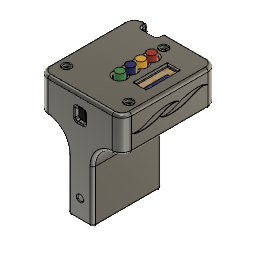
RangeFinderCase (Autodesk Fusion 360 design; units mm, degrees)
Autodesk Fusion 360 part; units mm, degrees
(part 1 of 2)
sketch "Sketch1" plane through (0, 0, 0) normal (0, 0, 1) x (1, 0, 0)
  line L0 (-22.5, 32.5) -> (22.5, 32.5) construction
  line L1 (22.5, 32.5) -> (22.5, -32.5) construction
  line L2 (22.5, -32.5) -> (-22.5, -32.5) construction
  line L3 (-22.5, -32.5) -> (-22.5, 32.5) construction
  circle A0 centre (-22.5, -32.5) radius 1.6
  circle A1 centre (-22.5, 32.5) radius 1.6 construction
  circle A2 centre (22.5, 32.5) radius 1.6 construction
  circle A3 centre (22.5, -32.5) radius 1.6
  line L4 (0, 32.5) -> (0, -32.5) construction
  circle A4 centre (-21.59, -29.21) radius 0.5 construction
  circle A5 centre (21.59, -29.21) radius 0.5 construction
  circle A6 centre (-21.59, 29.21) radius 0.5 construction
  circle A7 centre (21.59, 29.21) radius 0.5 construction
  line L5 (-21.59, 29.21) -> (-21.59, -29.21) construction
  line L6 (-21.59, -29.21) -> (21.59, -29.21) construction
  line L7 (21.59, -29.21) -> (21.59, 29.21) construction
  line L8 (21.59, 29.21) -> (-21.59, 29.21) construction
  line L9 (-21.59, 29.21) -> (21.59, -29.21) construction
  line L10 (21.59, 29.21) -> (-21.59, -29.21) construction
  circle A8 centre (1.27, 13.97) radius 1.6
  line L11 (25.25, 19.05) -> (-25.25, 19.05)
  line L12 (-25.25, 19.05) -> (-25.25, -35.25)
  line L13 (-25.25, -35.25) -> (25.25, -35.25)
  line L14 (25.25, -35.25) -> (25.25, 19.05)
  line L15 (25.25, 19.05) -> (-25.25, -35.25) construction
  line L16 (-25.25, 19.05) -> (25.25, -35.25) construction
  line L17 (-22.5, -32.5) -> (-25.25, -32.5) construction
  line L18 (-22.5, -32.5) -> (-22.5, -35.25) construction
  line L19 (20.32, 5.08) -> (12.7, 5.08)
  line L20 (12.7, 5.08) -> (12.7, -17.78)
  line L21 (12.7, -17.78) -> (20.32, -17.78)
  line L22 (20.32, -17.78) -> (20.32, 5.08)
  line L23 (16.51, 5.08) -> (16.51, -17.78) construction
  circle A9 centre (2.54, -19.05) radius 3.05
  circle A10 centre (2.54, -11.43) radius 3.05
  circle A11 centre (2.54, -3.81) radius 3.05
  circle A12 centre (2.54, 3.81) radius 3.05
  line L24 (2.54, -19.05) -> (2.54, -11.43) construction
  line L25 (2.54, -11.43) -> (2.54, -3.81) construction
  line L26 (2.54, -3.81) -> (2.54, 3.81) construction
  line L27 (-5.08, 17.78) -> (-22.86, 17.78)
  line L28 (-22.86, 17.78) -> (-22.86, -17.78)
  line L29 (-22.86, -17.78) -> (-5.08, -17.78)
  line L30 (-5.08, -17.78) -> (-5.08, 17.78)
  point P0 (0, -8.1)
  dimension "d15" = 45
  dimension "d16" = 65
  dimension "d18" = 3.2
  dimension "d47" = 58.42
  dimension "d48" = 43.18
  dimension "d49" = 1
  dimension "d50" = 43.18
  dimension "d51" = 22.86
  dimension "d52" = 50.5
  dimension "d53" = 5.08
  dimension "d68" = 7.62
  dimension "d69" = 22.86
  dimension "d71" = 11.43
  dimension "d74" = 6.1
  dimension "d75" = 7.62
  dimension "d76" = 10.16
  dimension "d80" = 17.78
  dimension "d81" = 35.56
  dimension "d83" = 11.43
  dimension "d182" = 1.27
  dimension "d188" = 1.27
  dimension "d189" = 19.05
  constraint horizontal L0
  constraint vertical L1
  constraint horizontal L2
  constraint vertical L3
  constraint coincident L2.end L3.start
  constraint coincident L0.start L3.end
  constraint coincident L0.end L1.start
  constraint coincident L1.end L2.start
  constraint equal A1 A2
  constraint equal A0 A1
  constraint equal A1 A3
  constraint midpoint L0 L4.start
  constraint midpoint L2 L4.end
  constraint midpoint origin L4
  constraint coincident A6.centre L5.start
  constraint coincident A4.centre L5.end
  constraint coincident A5.centre L6.end
  constraint coincident A7.centre L7.end
  constraint horizontal L8
  constraint vertical L5
  constraint equal L6 L8
  constraint equal L5 L7
  constraint midpoint origin L9
  constraint equal A6 A7
  constraint equal A4 A6
  constraint equal A5 A6
  constraint equal A1 A8
  constraint horizontal L11
  constraint perpendicular L11 L12
  constraint parallel L11 L13
  constraint parallel L12 L14
  constraint coincident L15 P0
  constraint coincident L16 P0
  constraint coincident L4 P0
  constraint coincident L12 L17.end
  constraint perpendicular L12 L17
  constraint coincident L13 L18.end
  constraint perpendicular L13 L18
  constraint equal L17 L18
  constraint horizontal L19
  constraint vertical L20
  constraint horizontal L21
  constraint vertical L22
  constraint midpoint L19 L23.start
  constraint midpoint L21 L23.end
  constraint coincident A9.centre L24.start
  constraint coincident A10.centre L24.end
  constraint vertical L24
  constraint coincident A11.centre L25.end
  constraint parallel L24 L25
  constraint coincident A12.centre L26.end
  constraint parallel L25 L26
  constraint equal L24 L25
  constraint equal L24 L26
  constraint equal A9 A10
  constraint equal A10 A11
  constraint equal A11 A12
  constraint horizontal L27
  constraint vertical L28
  constraint horizontal L29
  constraint vertical L30
  measures "d15" distance of L1.end L2.end
  measures "d16" distance of L0.start L2.end
  measures "d18" diameter of A1
  measures "d47" distance of A5.centre A7.centre
  measures "d48" distance of A4.centre A5.centre
  measures "d49" diameter of A6
  measures "d50" distance of L6 A8.centre
  measures "d51" distance of L5 A8.centre
  measures "d52" distance of L12.end L13.end
  measures "d53" distance of A8.centre L11
  measures "d68" distance of L19.start L19.end
  measures "d69" distance of L19.start L21.end
  measures "d71" distance of L6 L21
  measures "d74" diameter of A9
  measures "d75" distance of A9.centre A10.centre
  measures "d76" distance of L6 A9.centre
  measures "d80" distance of L28.end L29.end
  measures "d81" distance of L27.end L28.end
  measures "d83" distance of L6 L29
  measures "d182" distance of L7 L22
  measures "d188" distance of L5 L28
  measures "d189" distance of L7 L24
extrude "Extrude5" add sketch "Sketch1" along normal blind 1.2 contours L11 L12 L13 L14 | L19 L20 L21 L22 | A9 | A10 | A11 | A12 | L27 L28 L29 L30 makes body 1
sketch "Sketch5" plane through (0, -35.25, 0) normal (0, -1, 0) x (1, 0, 0)
  line L0 (-25.25, 0) -> (25.25, 0)
  line L1 (25.25, 0) -> (25.25, 1.2)
  line L2 (25.25, 1.2) -> (-25.25, 1.2)
  line L3 (-25.25, 1.2) -> (-25.25, 0)
  line L4 (13, 5.7) -> (-13, 5.7)
  line L5 (-13, 5.7) -> (-13, -12.3)
  line L6 (-13, -12.3) -> (13, -12.3)
  line L7 (13, -12.3) -> (13, 5.7)
  line L8 (13, 5.7) -> (-13, -12.3) construction
  line L9 (-13, 5.7) -> (13, -12.3) construction
  line L10 (0, -3.3) -> (0, 0) construction
  point P0 (0, -3.3)
  dimension "d56" = 26
  dimension "d57" = 18
  dimension "d58" = 4.5
  constraint horizontal L4
  constraint perpendicular L4 L5
  constraint parallel L4 L6
  constraint parallel L5 L7
  constraint coincident L8 P0
  constraint coincident L9 P0
  constraint coincident P0 L10.start
  constraint coincident L10.end origin
  constraint vertical L10
  measures "d56" distance of L4.start L4.end
  measures "d57" distance of L4.end L5.end
  measures "d58" distance of L2 L4
extrude "Extrude6" add sketch "Sketch5" along normal blind 5 contours L0 L2 L5 L7 | L0 L5 L6 L7 | L2 L4 L5 L7 bodies 1
sketch "Sketch6" plane through (0, -40.25, 0) normal (0, -1, 0) x (1, 0, 0)
  line L0 (13, -12.3) -> (13, 5.7)
  line L1 (13, 5.7) -> (-13, 5.7)
  line L2 (-13, 5.7) -> (-13, -12.3)
  line L3 (-13, -12.3) -> (13, -12.3)
  line L4 (0, 5.7) -> (0, -12.3) construction
  line L5 (-13, -3.3) -> (13, -3.3) construction
  line L6 (1.5, -0.8) -> (-1.5, -0.8)
  line L7 (-1.5, -0.8) -> (-1.5, -5.8)
  line L8 (-1.5, -5.8) -> (1.5, -5.8)
  line L9 (1.5, -5.8) -> (1.5, -0.8)
  line L10 (1.5, -0.8) -> (-1.5, -5.8) construction
  line L11 (-1.5, -0.8) -> (1.5, -5.8) construction
  point P0 (0, -3.3)
  dimension "d61" = 5
  dimension "d62" = 3
  constraint midpoint L1 L4.start
  constraint midpoint L3 L4.end
  constraint midpoint L2 L5.start
  constraint midpoint L0 L5.end
  constraint horizontal L6
  constraint perpendicular L6 L7
  constraint parallel L6 L8
  constraint parallel L7 L9
  constraint coincident L10 P0
  constraint coincident L11 P0
  constraint midpoint L4 P0
  measures "d61" distance of L6.start L8.end
  measures "d62" distance of L6.start L6.end
extrude "Extrude7" cut sketch "Sketch6" against normal blind 0.1 contours L6 L7 L8 L9 bodies 1
sketch "Sketch7" plane through (0, 0, 1.2) normal (0, 0, 1) x (-1, 0, 0)
  circle A0 centre (-1.27, -13.97) radius 1.6
  circle A1 centre (-22.5, 32.5) radius 1.6
  circle A2 centre (22.5, 32.5) radius 1.6
  line L0 (-25.25, 35.25) -> (-25.25, -19.05)
  line L1 (-25.25, -19.05) -> (25.25, -19.05)
  line L2 (25.25, -19.05) -> (25.25, 35.25)
  line L3 (25.25, 35.25) -> (13, 35.25)
  line L4 (13, 35.25) -> (-13, 35.25)
  line L5 (-13, 35.25) -> (-25.25, 35.25)
  circle A3 centre (-1.27, -13.97) radius 2.7
  circle A4 centre (22.5, 32.5) radius 2.7
  circle A5 centre (-22.5, 32.5) radius 2.7
  dimension "d65" = 5.4
  constraint concentric A0 A3
  constraint concentric A2 A4
  constraint concentric A1 A5
  constraint equal A4 A5
  constraint equal A3 A4
  measures "d65" diameter of A4
extrude "Extrude8" add sketch "Sketch7" along normal blind 6 contours A3 | A4 | A5 bodies 1
extrude "Extrude9" add sketch "Sketch1" along normal up to surface (3.7 mm away) contours L19 L20 L21 L22 bodies 1
extrude "Extrude10" add sketch "Sketch1" along normal up to surface (13.2 mm away) contours A9 | A10 | A11 | A12 bodies 1
extrude "Extrude11" add sketch "Sketch1" along normal up to surface (5.7 mm away) contours L27 L28 L29 L30 bodies 1
sketch "Sketch8" plane through (0, 17.78, 0) normal (0, 1, 0) x (-1, 0, 0)
  line L0 (5.08, 1.2) -> (22.86, 1.2)
  line L1 (22.86, 1.2) -> (22.86, 5.7)
  line L2 (22.86, 5.7) -> (5.08, 5.7)
  line L3 (5.08, 5.7) -> (5.08, 1.2)
  line L4 (18.47, 7.7) -> (9.47, 7.7)
  line L5 (9.47, 7.7) -> (9.47, 4.7)
  line L6 (9.47, 4.7) -> (18.47, 4.7)
  line L7 (18.47, 4.7) -> (18.47, 7.7)
  line L8 (18.47, 7.7) -> (9.47, 4.7) construction
  line L9 (9.47, 7.7) -> (18.47, 4.7) construction
  line L10 (13.97, 5.7) -> (13.97, 1.2) construction
  point P0 (13.97, 6.2)
  dimension "d86" = 3.5
  dimension "d87" = 9
  dimension "d88" = 3
  constraint horizontal L4
  constraint perpendicular L4 L5
  constraint parallel L4 L6
  constraint parallel L5 L7
  constraint coincident L8 P0
  constraint coincident L9 P0
  constraint midpoint L2 L10.start
  constraint midpoint L0 L10.end
  constraint coincident P0 L10
  measures "d86" distance of L0 L6
  measures "d87" distance of L4.start L4.end
  measures "d88" distance of L4.start L6.end
extrude "Extrude12" add sketch "Sketch8" along normal blind 0.5 and the other way blind 6 contours L2 L4 L5 L7 | L2 L5 L6 L7 bodies 1
sketch "Sketch9" plane through (0, 0, 0) normal (0, 0, -1) x (1, 0, 0)
  circle A0 centre (22.5, 32.5) radius 1.6
  circle A1 centre (1.27, -13.97) radius 1.6
  circle A2 centre (-22.5, 32.5) radius 1.6
  line L0 (25.25, -19.05) -> (25.25, 35.25)
  line L1 (25.25, 35.25) -> (13, 35.25)
  line L2 (13, 35.25) -> (-13, 35.25)
  line L3 (-13, 35.25) -> (-25.25, 35.25)
  line L4 (-25.25, 35.25) -> (-25.25, -19.05)
  line L5 (-25.25, -19.05) -> (25.25, -19.05)
  circle A3 centre (-22.5, 32.5) radius 2
  circle A4 centre (-22.5, 32.5) radius 4
  circle A5 centre (22.5, 32.5) radius 2
  circle A6 centre (22.5, 32.5) radius 4
  circle A7 centre (1.27, -13.97) radius 2
  circle A8 centre (1.27, -13.97) radius 4
  line L6 (27.25, -21.05) -> (-27.25, -21.05)
  line L7 (-27.25, -21.05) -> (-27.25, 42.25)
  line L8 (-27.25, 42.25) -> (27.25, 42.25)
  line L9 (27.25, 42.25) -> (27.25, -21.05)
  line L10 (0, -21.05) -> (0, -19.05) construction
  line L11 (27.25, 10.6) -> (25.25, 10.6) construction
  line L12 (-27.25, 10.6) -> (-25.25, 10.6) construction
  line L13 (0, 42.25) -> (0, 40.25) construction
  line L14 (-13, 40.25) -> (13, 40.25) construction
  dimension "d93" = 4
  dimension "d94" = 2
  dimension "d95" = 2
  constraint concentric A2 A3
  constraint concentric A3 A4
  constraint concentric A0 A5
  constraint concentric A0 A6
  constraint concentric A1 A7
  constraint concentric A7 A8
  constraint equal A3 A5
  constraint equal A3 A7
  constraint equal A4 A8
  constraint equal A4 A6
  constraint horizontal L6
  constraint vertical L7
  constraint horizontal L8
  constraint vertical L9
  constraint midpoint L6 L10.start
  constraint coincident L5 L10.end
  constraint perpendicular L5 L10
  constraint midpoint L9 L11.start
  constraint coincident L0 L11.end
  constraint perpendicular L0 L11
  constraint midpoint L7 L12.start
  constraint coincident L4 L12.end
  constraint perpendicular L4 L12
  constraint midpoint L8 L13.start
  constraint perpendicular L8 L13
  constraint coincident L13.end L14
  constraint equal L11 L13
  constraint equal L11 L12
  constraint equal L10 L11
  measures "d93" diameter of A3
  measures "d94" distance of A3 A4
  measures "d95" distance of L11.start L11.end
extrude "Extrude13" add sketch "Sketch9" along normal up to surface (13.3 mm away) separate body contours L0 L1 A6 | L0 L1 A6 | L3 L4 A4 | L3 L4 A4 | A8 makes body 2 at (26.4801, -32.8983, -8.8667) makes body 3 at (-18.5199, -32.8983, -8.8667) makes body 4 at (5.265, 14.1694, -8.8667)
sketch "Sketch10" plane through (0, 0, -13.3) normal (0, 0, -1) x (1, 0, 0)
  circle A0 centre (1.27, -13.97) radius 2
  circle A1 centre (1.27, -13.97) radius 4
  line L0 (28.25, -22.05) -> (-28.25, -22.05)
  line L1 (-28.25, -22.05) -> (-28.25, 43.25)
  line L2 (-28.25, 43.25) -> (28.25, 43.25)
  line L3 (28.25, 43.25) -> (28.25, -22.05)
  circle A2 centre (22.5, 32.5) radius 1.6
  circle A3 centre (1.27, -13.97) radius 1.6
  circle A4 centre (-22.5, 32.5) radius 1.6
  line L4 (25.25, -19.05) -> (25.25, 35.25)
  line L5 (25.25, 35.25) -> (13, 35.25)
  line L6 (13, 35.25) -> (-13, 35.25)
  line L7 (-13, 35.25) -> (-25.25, 35.25)
  line L8 (-25.25, 35.25) -> (-25.25, -19.05)
  line L9 (-25.25, -19.05) -> (25.25, -19.05)
  line L10 (-13, 35.25) -> (13, 35.25)
  line L11 (13, 35.25) -> (13, 40.25)
  line L12 (13, 40.25) -> (-13, 40.25)
  line L13 (-13, 40.25) -> (-13, 35.25)
  line L14 (28.25, 10.6) -> (25.25, 10.6) construction
  line L15 (-28.25, 10.6) -> (-25.25, 10.6) construction
  line L16 (0, -22.05) -> (0, -19.05) construction
  line L17 (0, 43.25) -> (0, 40.25) construction
  dimension "d98" = 3
  constraint horizontal L0
  constraint vertical L1
  constraint horizontal L2
  constraint vertical L3
  constraint midpoint L3 L14.start
  constraint coincident L4 L14.end
  constraint perpendicular L4 L14
  constraint midpoint L1 L15.start
  constraint coincident L8 L15.end
  constraint perpendicular L8 L15
  constraint midpoint L0 L16.start
  constraint coincident L9 L16.end
  constraint perpendicular L9 L16
  constraint midpoint L2 L17.start
  constraint coincident L12 L17.end
  constraint perpendicular L12 L17
  constraint equal L14 L16
  constraint equal L14 L17
  constraint equal L14 L15
  measures "d98" distance of L14.start L14.end
extrude "Extrude14" add sketch "Sketch10" along normal blind 2 contours A0 | A1 | L0 L1 L2 L3 | A2 | A3 | A4 | L4 L5 L6 L7 L8 L9 L10 | L6 L10 L11 L12 L13 bodies 2 3 4
fillet "Fillet4" radius 5 4 edges at (-28.25, -43.25, -14.3) (28.25, -43.25, -14.3) (28.25, 22.05, -14.3) (-28.25, 22.05, -14.3) on bodies 2
sketch "Sketch11" plane through (0, 0, -15.3) normal (0, 0, -1) x (1, 0, 0)
  line L0 (23.25, 43.25) -> (-23.25, 43.25)
  line L1 (-28.25, 38.25) -> (-28.25, -17.05)
  line L2 (-23.25, -22.05) -> (23.25, -22.05)
  line L3 (28.25, -17.05) -> (28.25, 38.25)
  arc A0 (-28.25, -17.05) -> (-23.25, -22.05) centre (-23.25, -17.05) ccw
  arc A1 (23.25, -22.05) -> (28.25, -17.05) centre (23.25, -17.05) ccw
  arc A2 (28.25, 38.25) -> (23.25, 43.25) centre (23.25, 38.25) ccw
  arc A3 (-23.25, 43.25) -> (-28.25, 38.25) centre (-23.25, 38.25) ccw
  line L4 (30.25, -17.05) -> (30.25, 38.25)
  arc A4 (30.25, 38.25) -> (23.25, 45.25) centre (23.25, 38.25) ccw
  line L5 (23.25, 45.25) -> (-23.25, 45.25)
  arc A5 (-23.25, 45.25) -> (-30.25, 38.25) centre (-23.25, 38.25) ccw
  line L6 (-30.25, 38.25) -> (-30.25, -17.05)
  arc A6 (-30.25, -17.05) -> (-23.25, -24.05) centre (-23.25, -17.05) ccw
  line L7 (-23.25, -24.05) -> (23.25, -24.05)
  arc A7 (23.25, -24.05) -> (30.25, -17.05) centre (23.25, -17.05) ccw
  dimension "d101" = 2
extrude "Extrude15" add sketch "Sketch11" against normal up to surface (23.5 mm away) bodies 2
sketch "Sketch12" plane through (0, 24.05, 0) normal (0, 1, 0) x (-1, 0, 0)
  line L0 (23.25, 8.2) -> (-23.25, 8.2)
  line L1 (-23.25, 8.2) -> (-23.25, -15.3)
  line L2 (-23.25, -15.3) -> (23.25, -15.3)
  line L3 (23.25, -15.3) -> (23.25, 8.2)
  line L4 (9.47, 4.7) -> (18.47, 4.7)
  line L5 (18.47, 4.7) -> (18.47, 7.7)
  line L6 (18.47, 7.7) -> (9.47, 7.7)
  line L7 (9.47, 7.7) -> (9.47, 4.7)
  line L8 (9.47, 7.7) -> (18.47, 4.7) construction
  line L9 (18.47, 7.7) -> (9.47, 4.7) construction
  line L10 (19.97, 9.45) -> (7.97, 9.45)
  line L11 (7.97, 9.45) -> (7.97, 2.95)
  line L12 (7.97, 2.95) -> (19.97, 2.95)
  line L13 (19.97, 2.95) -> (19.97, 9.45)
  line L14 (19.97, 9.45) -> (7.97, 2.95) construction
  line L15 (7.97, 9.45) -> (19.97, 2.95) construction
  point P0 (13.97, 6.2)
  point P1 (13.97, 6.2)
  dimension "d106" = 6.5
  dimension "d107" = 12
  constraint coincident L6.end L7.start
  constraint coincident L4.end L5.start
  constraint coincident L5.end L6.start
  constraint coincident L4.start L7.end
  constraint coincident L8 P1
  constraint coincident L9 P1
  constraint horizontal L10
  constraint perpendicular L10 L11
  constraint parallel L10 L12
  constraint parallel L11 L13
  constraint coincident L14 P1
  constraint coincident L15 P1
  constraint coincident P1 P0
  measures "d106" distance of L10.start L12.end
  measures "d107" distance of L11.end L12.end
extrude "Extrude16" cut sketch "Sketch12" against normal blind 2 contours L0 L11 L12 L13 | L0 L10 L11 L13 | L4 L5 L6 L7 bodies 2
fillet "Fillet5" radius 2 2 edges at (-19.97, 23.05, 2.95) (-7.97, 23.05, 2.95) on bodies 2
sketch "Sketch13" plane through (0, 0, 8.2) normal (0, 0, 1) x (-1, 0, 0)
  line L0 (-23.25, 43.25) -> (23.25, 43.25)
  arc A0 (28.25, 38.25) -> (23.25, 43.25) centre (23.25, 38.25) ccw
  line L1 (28.25, 38.25) -> (28.25, -17.05)
  arc A1 (23.25, -22.05) -> (28.25, -17.05) centre (23.25, -17.05) ccw
  line L2 (7.97, -22.05) -> (-23.25, -22.05)
  arc A2 (-28.25, -17.05) -> (-23.25, -22.05) centre (-23.25, -17.05) ccw
  line L3 (-28.25, -17.05) -> (-28.25, 38.25)
  arc A3 (-23.25, 43.25) -> (-28.25, 38.25) centre (-23.25, 38.25) ccw
  line L4 (-30.25, 38.25) -> (-30.25, -17.05)
  arc A4 (-30.25, -17.05) -> (-23.25, -24.05) centre (-23.25, -17.05) ccw
  line L5 (19.97, -24.05) -> (23.25, -24.05)
  arc A5 (23.25, -24.05) -> (30.25, -17.05) centre (23.25, -17.05) ccw
  line L6 (30.25, -17.05) -> (30.25, 38.25)
  arc A6 (30.25, 38.25) -> (23.25, 45.25) centre (23.25, 38.25) ccw
  line L7 (23.25, 45.25) -> (-23.25, 45.25)
  arc A7 (-23.25, 45.25) -> (-30.25, 38.25) centre (-23.25, 38.25) ccw
  line L8 (-12.7, 17.78) -> (-20.32, 17.78)
  line L9 (-20.32, 17.78) -> (-20.32, -5.08)
  line L10 (-20.32, -5.08) -> (-12.7, -5.08)
  line L11 (-12.7, -5.08) -> (-12.7, 17.78)
  circle A8 centre (-2.54, 19.05) radius 3.05 construction
  circle A9 centre (-2.54, 11.43) radius 3.05 construction
  circle A10 centre (-2.54, 3.81) radius 3.05 construction
  circle A11 centre (-2.54, -3.81) radius 3.05 construction
  circle A12 centre (-2.54, 19.05) radius 4.06
  circle A13 centre (-2.54, 11.43) radius 4.06
  circle A14 centre (-2.54, 3.81) radius 4.06
  circle A15 centre (-2.54, -3.81) radius 4.06
  line L12 (-2.54, 15.49) -> (-2.54, 14.99) construction
  line L13 (19.97, -22.05) -> (19.97, -24.05)
  line L14 (-23.25, -24.05) -> (7.97, -24.05)
  line L15 (7.97, -24.05) -> (7.97, -22.05)
  line L16 (23.25, -22.05) -> (19.97, -22.05)
  line L17 (11.2, -21.95) -> (-23.25, -21.95)
  arc A16 (-28.15, -17.05) -> (-23.25, -21.95) centre (-23.25, -17.05) ccw
  line L18 (-28.15, -17.05) -> (-28.15, 38.25)
  arc A17 (-23.25, 43.15) -> (-28.15, 38.25) centre (-23.25, 38.25) ccw
  line L19 (-23.25, 43.15) -> (23.25, 43.15)
  arc A18 (28.15, 38.25) -> (23.25, 43.15) centre (23.25, 38.25) ccw
  line L20 (28.15, 38.25) -> (28.15, -17.05)
  arc A19 (23.25, -21.95) -> (28.15, -17.05) centre (23.25, -17.05) ccw
  line L21 (8.38, -20.05) -> (-23.25, -20.05)
  arc A20 (-26.25, -17.05) -> (-23.25, -20.05) centre (-23.25, -17.05) ccw
  line L22 (-26.25, -17.05) -> (-26.25, 38.25)
  arc A21 (-23.25, 41.25) -> (-26.25, 38.25) centre (-23.25, 38.25) ccw
  line L23 (-23.25, 41.25) -> (23.25, 41.25)
  arc A22 (26.25, 38.25) -> (23.25, 41.25) centre (23.25, 38.25) ccw
  line L24 (26.25, 38.25) -> (26.25, -17.05)
  arc A23 (23.25, -20.05) -> (26.25, -17.05) centre (23.25, -17.05) ccw
  line L25 (8.38, -20.05) -> (23.25, -20.05)
  line L26 (11.2, -21.95) -> (23.25, -21.95)
  line L27 (7.97, -24.05) -> (19.97, -24.05)
  line L28 (7.97, -22.05) -> (19.97, -22.05)
  line L29 (9.47, -18.28) -> (18.47, -18.28)
  line L30 (18.47, -18.28) -> (18.47, -11.78)
  line L31 (18.47, -11.78) -> (9.47, -11.78)
  line L32 (9.47, -11.78) -> (9.47, -18.28)
  line L33 (7.97, -22.05) -> (7.97, -18.28)
  line L34 (7.97, -18.28) -> (9.47, -18.28)
  line L35 (19.97, -22.05) -> (19.97, -18.28)
  line L36 (19.97, -18.28) -> (18.47, -18.28)
  dimension "d112" = -0.1
  dimension "d113" = -2
  dimension "d116" = 0.5
  constraint equal A12 A13
  constraint equal A12 A14
  constraint equal A12 A15
  constraint coincident A13 L12.start
  constraint coincident A12 L12.end
  constraint vertical L12
  constraint coincident A8.centre L12
  constraint horizontal L25
  constraint parallel L25 L26
  constraint coincident L21.start L25.start
  constraint coincident A23.start L25.end
  constraint coincident A19.start L26.end
  constraint perpendicular L15 L27
  constraint coincident L14.end L15.start
  constraint coincident L5.start L13.end
  constraint coincident L2.start L15.end
  constraint coincident L13.start L16.end
  constraint coincident L29.start L32.end
  constraint coincident L29.end L30.start
  constraint vertical L33
  constraint vertical L35
  constraint horizontal L36
  constraint horizontal L34
  constraint coincident L17.start L26.start
  constraint concentric A8 A12
  constraint concentric A9 A13
  constraint concentric A10 A14
  constraint concentric A11 A15
  measures "d116" distance of L12.start L12.end
extrude "Extrude17" add sketch "Sketch13" along normal blind 2 separate body contours L0 A0 L1 A1 L2 A2 L3 A3 L4 A4 L5 A5 L6 A6 L7 A7 L13 L14 L15 L16 | L0 A0 L1 A1 L2 A2 L3 A3 L16 L17 A16 L18 A17 L19 A18 L20 A19 L26 L33 L35 | L17 A16 L18 A17 L19 A18 L20 A19 L21 A20 L22 A21 L23 A22 L24 A23 L25 L26 L33 L35 | L21 A20 L22 A21 L23 A22 L24 A23 L25 L30 L31 L32 L33 L34 L35 L36 | L29 L30 L31 L32 makes body 5
fillet "Fillet6" radius 0.5 6 edges at (3.9427, -15.24, 9.2) (1.1373, -15.24, 9.2) (3.9427, -7.62, 9.2) (1.1373, -7.62, 9.2) (3.9427, 0, 9.2) (1.1373, 0, 9.2) on bodies 5
extrude "Extrude18" add sketch "Sketch13" against normal blind 1 contours L17 A16 L18 A17 L19 A18 L20 A19 L21 A20 L22 A21 L23 A22 L24 A23 L25 L26 L33 L35 bodies 5
fillet "Fillet7" radius 2 2 edges at (-7.97, 18.28, 9.2) (-19.97, 18.28, 9.2) on bodies 5
sketch "Sketch14" plane through (0, -43.25, 0) normal (0, 1, 0) x (-1, 0, 0)
  line L0 (-23.25, -13.3) -> (23.25, -13.3)
  line L1 (23.25, -13.3) -> (23.25, 8.2)
  line L2 (23.25, 8.2) -> (-23.25, 8.2)
  line L3 (-23.25, 8.2) -> (-23.25, -13.3)
  line L4 (1.5, -0.8) -> (-1.5, -0.8)
  line L5 (-1.5, -0.8) -> (-1.5, -5.8)
  line L6 (-1.5, -5.8) -> (1.5, -5.8)
  line L7 (1.5, -5.8) -> (1.5, -0.8)
  line L8 (-13, -12.3) -> (-13, 5.7)
  line L9 (-13, 5.7) -> (13, 5.7)
  line L10 (13, 5.7) -> (13, -12.3)
  line L11 (13, -12.3) -> (-13, -12.3)
  line L12 (3, -7.3) -> (3, 0.7)
  line L13 (3, 0.7) -> (-3, 0.7)
  line L14 (-3, 0.7) -> (-3, -7.3)
  line L15 (-3, -7.3) -> (3, -7.3)
  dimension "d123" = 1.5
extrude "Extrude19" cut sketch "Sketch14" against normal blind 2 draft 27 contours L4 L5 L6 L7 | L12 L13 L14 L15 bodies 2
fillet "Fillet8" radius 2 4 edges at (-3.5095, -44.25, 1.2095) (3.5095, -44.25, 1.2095) (3.5095, -44.25, -7.8095) (-3.5095, -44.25, -7.8095) on bodies 2
fillet "Fillet9" radius 1 8 edges at (3.5175, -45.25, 1.2175) (0, -45.25, 1.7191) (-3.5175, -45.25, 1.2175) (-4.0191, -45.25, -3.3) (-3.5175, -45.25, -7.8175) (0, -45.25, -8.3191) (3.5175, -45.25, -7.8175) (4.0191, -45.25, -3.3) on bodies 2
fillet "Fillet11" radius 1 16 edges at (0.5345, -15.24, 10.2) (-1.52, -11.43, 10.2) (0.5345, -7.62, 10.2) (-1.52, -3.81, 10.2) (0.5345, 0, 10.2) (2.54, 7.87, 10.2) (4.5455, 0, 10.2) (6.6, -3.81, 10.2) (4.5455, -7.62, 10.2) (6.6, -11.43, 10.2) (4.5455, -15.24, 10.2) (2.54, -23.11, 10.2) (16.51, -17.78, 10.2) (12.7, -6.35, 10.2) (16.51, 5.08, 10.2) (20.32, -6.35, 10.2) on bodies 5
fillet "Fillet15" radius 2 9 edges at (-21.61, 24.05, 10.2) (-28.1997, 21.9997, 10.2) (-30.25, -10.6, 10.2) (-28.1997, -43.1997, 10.2) (0, -45.25, 10.2) (28.1997, -43.1997, 10.2) (30.25, -10.6, 10.2) (28.1997, 21.9997, 10.2) (7.64, 24.05, 10.2) on bodies 5
sketch "Sketch15" plane through (0, -45.25, 0) normal (0, -1, 0) x (1, 0, 0)
  line L0 (23.25, 8.2) -> (-23.25, 8.2)
  line L1 (-23.25, 8.2) -> (-23.25, -15.3)
  line L2 (-23.25, -15.3) -> (23.25, -15.3)
  line L3 (23.25, -15.3) -> (23.25, 8.2)
  ellipse E0 centre (1.2649, -1.0351) end of major axis (3.8796, 1.5796) minor radius 3 (4.6319, -0.3412) -> (1.9588, 2.3319) ccw
  line L4 (4.6319, -0.3412) -> (4.6319, -6.2588)
  ellipse E1 centre (1.2649, -5.5649) end of major axis (3.8796, -8.1796) minor radius 3 (1.9588, -8.9319) -> (4.6319, -6.2588) ccw
  line L5 (1.9588, -8.9319) -> (-1.9588, -8.9319)
  ellipse E2 centre (-1.2649, -5.5649) end of major axis (-3.8796, -8.1796) minor radius 3 (-4.6319, -6.2588) -> (-1.9588, -8.9319) ccw
  line L6 (-4.6319, -6.2588) -> (-4.6319, -0.3412)
  ellipse E3 centre (-1.2649, -1.0351) end of major axis (-3.8796, 1.5796) minor radius 3 (-1.9588, 2.3319) -> (-4.6319, -0.3412) ccw
  line L7 (-1.9588, 2.3319) -> (1.9588, 2.3319)
  line L8 (-8, -15.3) -> (8, -15.3)
  line L9 (8, -15.3) -> (8, -69.75)
  line L10 (8, -69.75) -> (-8, -69.75)
  line L11 (-8, -69.75) -> (-8, -15.3)
  line L12 (0, 8.2) -> (0, -15.3) construction
  circle A0 centre (0, -48.025) radius 2.725
  circle A1 centre (0, -62.025) radius 2.725
  line L13 (0, -48.025) -> (0, -62.025) construction
  line L14 (0, -15.3) -> (0, -48.025) construction
  line L15 (-8, -64.75) -> (8, -64.75) construction
  line L16 (-8, -45.3) -> (8, -45.3) construction
  circle A2 centre (0, -55.025) radius 2.1
  dimension "d134" = 16
  dimension "d135" = 14
  dimension "d136" = 5.45
  dimension "d137" = 5
  dimension "d138" = 30
  dimension "d139" = 4.2
  constraint horizontal L8
  constraint vertical L9
  constraint horizontal L10
  constraint vertical L11
  constraint coincident L2 L8.start
  constraint midpoint L0 L12.start
  constraint midpoint L2 L12.end
  constraint midpoint L8 L12.end
  constraint coincident A0.centre L13.start
  constraint coincident A1.centre L13.end
  constraint equal A0 A1
  constraint vertical L14
  constraint vertical L13
  constraint coincident L11 L15.start
  constraint coincident L9 L15.end
  constraint perpendicular L9 L15
  constraint tangent A1 L15
  constraint coincident L11 L16.start
  constraint coincident L9 L16.end
  constraint perpendicular L9 L16
  constraint tangent A0 L16
  constraint midpoint L13 A2.centre
  measures "d134" distance of L8.start L8.end
  measures "d135" vertical distance of A0.centre A1.centre
  measures "d136" diameter of A0
  measures "d137" distance of L10 L15
  measures "d138" distance of L8 L16
  measures "d139" diameter of A2
extrude "Extrude20" add sketch "Sketch15" against normal blind 25 contours L2 L8 L9 L10 L11 | A0 | A1 | A2 bodies 2
extrude "Extrude21" cut sketch "Sketch15" against normal blind 20 contours A2 bodies 2
extrude "Extrude22" cut sketch "Sketch15" along normal blind 10 from surface at -25 contours A0 | A1 bodies 2
sketch "Sketch16" plane through (0, 0, -15.3) normal (0, 0, -1) x (1, 0, 0)
  line L0 (-8, 20.25) -> (-8, 45.25)
  line L1 (-8, 45.25) -> (-23.25, 45.25)
  arc A0 (-23.25, 45.25) -> (-30.25, 38.25) centre (-23.25, 38.25) ccw
  line L2 (-30.25, 38.25) -> (-30.25, -17.05)
  arc A1 (-30.25, -17.05) -> (-23.25, -24.05) centre (-23.25, -17.05) ccw
  line L3 (-23.25, -24.05) -> (23.25, -24.05)
  arc A2 (23.25, -24.05) -> (30.25, -17.05) centre (23.25, -17.05) ccw
  line L4 (30.25, -17.05) -> (30.25, 38.25)
  arc A3 (30.25, 38.25) -> (23.25, 45.25) centre (23.25, 38.25) ccw
  line L5 (23.25, 45.25) -> (8, 45.25)
  line L6 (8, 45.25) -> (8, 20.25)
  line L7 (8, 20.25) -> (-8, 20.25)
  line L8 (-5.2, 20.25) -> (5.2, 20.25)
  line L9 (5.2, 20.25) -> (5.2, -4.75)
  line L10 (5.2, -4.75) -> (-5.2, -4.75)
  line L11 (-5.2, -4.75) -> (-5.2, 20.25)
  line L12 (0, 20.25) -> (0, 0) construction
  line L13 (5.2, -4.75) -> (9.2, -4.75)
  line L14 (9.2, -4.75) -> (9.2, 45.25)
  line L15 (-5.2, -4.75) -> (-9.2, -4.75)
  line L16 (-9.2, -4.75) -> (-9.2, 45.25)
  dimension "d147" = 10.4
  dimension "d148" = 25
  dimension "d149" = 4
  constraint horizontal L8
  constraint vertical L9
  constraint horizontal L10
  constraint vertical L11
  constraint coincident L7 L8.start
  constraint midpoint L7 L12.start
  constraint coincident L12.end origin
  constraint midpoint L8 L12.start
  constraint perpendicular L9 L13
  constraint coincident L5 L14.end
  constraint perpendicular L5 L14
  constraint perpendicular L11 L15
  constraint coincident L1 L16.end
  constraint perpendicular L1 L16
  constraint equal L13 L15
  measures "d147" distance of L9.end L10.end
  measures "d148" distance of L8.end L9.end
  measures "d149" distance of L9 L14
extrude "Extrude23" add sketch "Sketch16" along normal up to surface (54.45 mm away) contours L0 L1 L7 L11 L15 L16 | L5 L6 L7 L9 L13 L14 bodies 2
sketch "Sketch20" plane through (0, -20.25, 0) normal (0, 1, 0) x (-1, 0, 0)
  circle A0 centre (0, -62.025) radius 2.725
  circle A1 centre (0, -48.025) radius 2.725
  line L0 (-5.2, -15.3) -> (-5.2, -69.75)
  line L1 (-5.2, -69.75) -> (5.2, -69.75)
  line L2 (5.2, -69.75) -> (5.2, -15.3)
  line L3 (5.2, -15.3) -> (-5.2, -15.3)
  line L4 (-5.2, -45.3) -> (5.2, -45.3) construction
  line L5 (-5.2, -41.2) -> (5.2, -41.2)
  dimension "d185" = 4.1
  constraint coincident L0 L4.start
  constraint coincident L2 L4.end
  constraint perpendicular L2 L4
  constraint tangent A1 L4
  constraint coincident L0 L5.start
  constraint coincident L2 L5.end
  constraint perpendicular L2 L5
  measures "d185" distance of L4 L5
extrude "Extrude28" add sketch "Sketch20" along normal up to surface (25 mm away) contours L0 L2 L3 L5 bodies 2
fillet "Fillet12" radius 16 3 edges at (-9.2, -20.25, -15.3) (9.2, -20.25, -15.3) (0, 4.75, -15.3) on bodies 2
fillet "Fillet13" radius 2 4 edges at (5.2, -20.25, -42.525) (-5.2, -20.25, -42.525) (5.2, 4.75, -42.525) (-5.2, 4.75, -42.525) on bodies 2
fillet "Fillet14" radius 2 18 edges at (-9.2, -45.25, -50.525) (-13.2167, -45.25, -20.6981) (-24.2204, -45.1818, -15.3304) (-28.8469, -42.4542, -15.3) (-30.25, -10.6, -15.3) (-28.1997, 21.9997, -15.3) (0, 24.05, -15.3) (28.1997, 21.9997, -15.3) (30.25, -10.6, -15.3) (28.8469, -42.4542, -15.3) (24.2204, -45.1818, -15.3304) (13.2167, -45.25, -20.6981) (9.2, -45.25, -50.525) (-9.2, 4.75, -50.525) (-13.8863, 9.4363, -19.9863) (9.2, 4.75, -50.525) (13.8863, 9.4363, -19.9863) (0, 4.75, -41.2) on bodies 2
fillet "Fillet16" radius 2 12 edges at (5.2, -7.75, -69.75) (4.6142, -19.6642, -69.75) (0, -20.25, -69.75) (-4.6142, -19.6642, -69.75) (-5.2, -7.75, -69.75) (-7.2, 4.75, -69.75) (-9.2, -20.25, -69.75) (-8.6171, -44.6671, -69.75) (0, -45.25, -69.75) (8.6171, -44.6671, -69.75) (9.2, -20.25, -69.75) (7.2, 4.75, -69.75) on bodies 2
fillet "Fillet17" radius 0.5 3 edges at (-2.5406, -20.25, -49.0104) (-2.5406, -20.25, -63.0104) (-1.9579, -45.25, -54.2656) on bodies 2
fillet "Fillet18" radius 1 12 edges at (-7.97, 24.05, 6.575) (-8.5558, 24.05, 3.5358) (-13.97, 24.05, 2.95) (-19.3842, 24.05, 3.5358) (-19.97, 24.05, 6.575) (-7.97, 23.4642, 9.6142) (-7.97, 21.165, 10.2) (-8.5558, 18.8658, 10.2) (-13.97, 18.28, 10.2) (-19.3842, 18.8658, 10.2) (-19.97, 21.165, 10.2) (-19.97, 23.4642, 9.6142) on bodies 2 5
sketch "Sketch17" plane through (0, 0, 8.2) normal (0, 0, -1) x (1, 0, 0)
  line L0 (-23.25, -20.05) -> (-19.9567, -20.05)
  arc A0 (-17.97, -18.28) -> (-19.9567, -20.05) centre (-17.97, -20.28) ccw
  line L1 (-17.97, -18.28) -> (-9.97, -18.28)
  arc A1 (-7.9833, -20.05) -> (-9.97, -18.28) centre (-9.97, -20.28) ccw
  line L2 (-7.9833, -20.05) -> (23.25, -20.05)
  arc A2 (23.25, -20.05) -> (26.25, -17.05) centre (23.25, -17.05) ccw
  line L3 (26.25, -17.05) -> (26.25, 38.25)
  arc A3 (26.25, 38.25) -> (23.25, 41.25) centre (23.25, 38.25) ccw
  line L4 (23.25, 41.25) -> (-23.25, 41.25)
  arc A4 (-23.25, 41.25) -> (-26.25, 38.25) centre (-23.25, 38.25) ccw
  line L5 (-26.25, 38.25) -> (-26.25, -17.05)
  arc A5 (-26.25, -17.05) -> (-23.25, -20.05) centre (-23.25, -17.05) ccw
  arc A6 (0.3092, -0.4178) -> (0.3092, 0.4178) centre (0.0345, 0) ccw
  arc A7 (0.3092, 7.2022) -> (0.3092, 0.4178) centre (2.54, 3.81) ccw
  arc A8 (0.3092, 7.2022) -> (0.3092, 8.0378) centre (0.0345, 7.62) ccw
  arc A9 (0.3092, 14.8222) -> (0.3092, 8.0378) centre (2.54, 11.43) ccw
  arc A10 (0.3092, 14.8222) -> (0.3092, 15.6578) centre (0.0345, 15.24) ccw
  arc A11 (4.7708, 15.6578) -> (0.3092, 15.6578) centre (2.54, 19.05) ccw
  arc A12 (4.7708, 15.6578) -> (4.7708, 14.8222) centre (5.0455, 15.24) ccw
  arc A13 (4.7708, 8.0378) -> (4.7708, 14.8222) centre (2.54, 11.43) ccw
  arc A14 (4.7708, 8.0378) -> (4.7708, 7.2022) centre (5.0455, 7.62) ccw
  arc A15 (0.3092, -0.4178) -> (4.7708, -0.4178) centre (2.54, -3.81) ccw
  line L6 (12.7, -5.08) -> (12.7, 17.78)
  line L7 (12.7, 17.78) -> (20.32, 17.78)
  line L8 (20.32, 17.78) -> (20.32, -5.08)
  line L9 (20.32, -5.08) -> (12.7, -5.08)
  circle A16 centre (-22.5, 32.5) radius 1.6
  circle A17 centre (-22.5, 32.5) radius 2.7
  circle A18 centre (22.5, 32.5) radius 1.6
  circle A19 centre (22.5, 32.5) radius 2.7
  circle A20 centre (1.27, -13.97) radius 1.6
  circle A21 centre (1.27, -13.97) radius 2.7
  circle A22 centre (-22.5, 32.5) radius 3.75
  circle A23 centre (22.5, 32.5) radius 3.75
  circle A24 centre (1.27, -13.97) radius 3.75
  arc A25 (4.7708, 0.4178) -> (4.7708, 7.2022) centre (2.54, 3.81) ccw
  arc A26 (4.7708, 0.4178) -> (4.7708, -0.4178) centre (5.0455, 0) ccw
  constraint concentric A16 A22
  constraint concentric A18 A23
  constraint concentric A20 A24
  constraint equal A22 A24
  constraint equal A22 A23
  constraint tangent L5 A22
extrude "Extrude24" cut sketch "Sketch17" against normal up to surface (2 mm away) contours A16 | A18 | A20 bodies 5
extrude "Extrude25" add sketch "Sketch17" along normal up to surface (1 mm away) contours A23 | A22 | A17 | A19 | A21 | A24 bodies 5
sketch "Sketch18" plane through (0, 0, 10.2) normal (0, 0, 1) x (-1, 0, 0)
  circle A0 centre (-22.5, 32.5) radius 1.6
  circle A1 centre (22.5, 32.5) radius 1.6
  circle A2 centre (-1.27, -13.97) radius 1.6
  line L0 (20.97, -20.28) -> (20.97, -22.05)
  line L1 (20.97, -22.05) -> (23.25, -22.05)
  arc A3 (23.25, -22.05) -> (28.25, -17.05) centre (23.25, -17.05) ccw
  line L2 (28.25, -17.05) -> (28.25, 38.25)
  arc A4 (28.25, 38.25) -> (23.25, 43.25) centre (23.25, 38.25) ccw
  line L3 (23.25, 43.25) -> (-23.25, 43.25)
  arc A5 (-23.25, 43.25) -> (-28.25, 38.25) centre (-23.25, 38.25) ccw
  line L4 (-28.25, 38.25) -> (-28.25, -17.05)
  arc A6 (-28.25, -17.05) -> (-23.25, -22.05) centre (-23.25, -17.05) ccw
  line L5 (-23.25, -22.05) -> (6.97, -22.05)
  line L6 (6.97, -22.05) -> (6.97, -20.28)
  arc A7 (9.97, -17.28) -> (6.97, -20.28) centre (9.97, -20.28) ccw
  line L7 (9.97, -17.28) -> (17.97, -17.28)
  arc A8 (20.97, -20.28) -> (17.97, -17.28) centre (17.97, -20.28) ccw
  arc A9 (0.7898, 15.24) -> (-5.8698, 15.24) centre (-2.54, 19.05) ccw
  arc A10 (0.7898, 7.62) -> (0.7898, 15.24) centre (-2.54, 11.43) ccw
  arc A11 (0.7898, 0) -> (0.7898, 7.62) centre (-2.54, 3.81) ccw
  arc A12 (-5.8698, 0) -> (0.7898, 0) centre (-2.54, -3.81) ccw
  line L8 (-11.7, 18.78) -> (-11.7, -6.08)
  line L9 (-11.7, -6.08) -> (-21.32, -6.08)
  line L10 (-21.32, -6.08) -> (-21.32, 18.78)
  line L11 (-21.32, 18.78) -> (-11.7, 18.78)
  circle A13 centre (-22.5, 32.5) radius 2.75
  circle A14 centre (22.5, 32.5) radius 2.75
  circle A15 centre (-1.27, -13.97) radius 2.75
  arc A16 (-5.8698, 7.62) -> (-5.8698, 0) centre (-2.54, 3.81) ccw
  arc A17 (-5.8698, 15.24) -> (-5.8698, 7.62) centre (-2.54, 11.43) ccw
  dimension "d172" = 5.5
  constraint concentric A0 A13
  constraint concentric A1 A14
  constraint concentric A2 A15
  constraint equal A13 A14
  constraint equal A13 A15
  measures "d172" diameter of A13
extrude "Extrude26" cut sketch "Sketch18" against normal blind 2 contours A13 | A14 | A15 bodies 5
fillet "Fillet19" radius 0.5 3 edges at (3.8339, 12.9756, 10.2) (25.0639, -33.4944, 10.2) (-19.9361, -33.4944, 10.2) on bodies 5
sketch "Sketch19" plane through (0, 0, 8.2) normal (0, 0, -1) x (1, 0, 0)
  circle A0 centre (1.27, -13.97) radius 3.75
  line L0 (-23.25, -20.05) -> (-19.9567, -20.05)
  arc A1 (-17.97, -18.28) -> (-19.9567, -20.05) centre (-17.97, -20.28) ccw
  line L1 (-17.97, -18.28) -> (-9.97, -18.28)
  arc A2 (-7.9833, -20.05) -> (-9.97, -18.28) centre (-9.97, -20.28) ccw
  line L2 (-7.9833, -20.05) -> (23.25, -20.05)
  arc A3 (23.25, -20.05) -> (26.25, -17.05) centre (23.25, -17.05) ccw
  line L3 (26.25, -17.05) -> (26.25, 32.5)
  circle A4 centre (22.5, 32.5) radius 3.75
  line L4 (26.25, 32.5) -> (26.25, 38.25)
  arc A5 (26.25, 38.25) -> (23.25, 41.25) centre (23.25, 38.25) ccw
  line L5 (23.25, 41.25) -> (-23.25, 41.25)
  arc A6 (-23.25, 41.25) -> (-26.25, 38.25) centre (-23.25, 38.25) ccw
  line L6 (-26.25, 38.25) -> (-26.25, 32.5)
  circle A7 centre (-22.5, 32.5) radius 3.75
  line L7 (-26.25, 32.5) -> (-26.25, -17.05)
  arc A8 (-26.25, -17.05) -> (-23.25, -20.05) centre (-23.25, -17.05) ccw
  arc A9 (0.3092, -0.4178) -> (0.3092, 0.4178) centre (0.0345, 0) ccw
  arc A10 (0.3092, 7.2022) -> (0.3092, 0.4178) centre (2.54, 3.81) ccw
  arc A11 (0.3092, 7.2022) -> (0.3092, 8.0378) centre (0.0345, 7.62) ccw
  arc A12 (0.3092, 14.8222) -> (0.3092, 8.0378) centre (2.54, 11.43) ccw
  arc A13 (0.3092, 14.8222) -> (0.3092, 15.6578) centre (0.0345, 15.24) ccw
  arc A14 (4.7708, 15.6578) -> (0.3092, 15.6578) centre (2.54, 19.05) ccw
  arc A15 (4.7708, 15.6578) -> (4.7708, 14.8222) centre (5.0455, 15.24) ccw
  arc A16 (4.7708, 8.0378) -> (4.7708, 14.8222) centre (2.54, 11.43) ccw
  arc A17 (4.7708, 8.0378) -> (4.7708, 7.2022) centre (5.0455, 7.62) ccw
  arc A18 (0.3092, -0.4178) -> (4.7708, -0.4178) centre (2.54, -3.81) ccw
  line L8 (12.7, -5.08) -> (12.7, 17.78)
  line L9 (12.7, 17.78) -> (20.32, 17.78)
  line L10 (20.32, 17.78) -> (20.32, -5.08)
  line L11 (20.32, -5.08) -> (12.7, -5.08)
  line L12 (-9.47, -11.78) -> (-9.47, -18.28)
  line L13 (-9.47, -18.28) -> (-18.47, -18.28)
  line L14 (-18.47, -18.28) -> (-18.47, -11.78)
  line L15 (-18.47, -11.78) -> (-9.47, -11.78)
  arc A19 (4.7708, 0.4178) -> (4.7708, 7.2022) centre (2.54, 3.81) ccw
  arc A20 (4.7708, 0.4178) -> (4.7708, -0.4178) centre (5.0455, 0) ccw
  line L16 (-9.47, -18.28) -> (-9.47, -24.05)
  line L17 (-18.47, -18.28) -> (-18.47, -24.05)
  line L18 (-18.47, -24.05) -> (-9.47, -24.05)
  line L19 (23.25, -24.05) -> (-6.97, -24.05)
  constraint coincident L12.end L13.start
  constraint perpendicular L13 L16
  constraint coincident L13.end L14.start
  constraint perpendicular L13 L17
  constraint horizontal L18
  constraint coincident L16.end L19
extrude "Extrude27" cut sketch "Sketch19" against normal blind 1 contours A1 L13 L17 | A1 L1 A2 L13 L16 L17 L18 | L1 L12 L13 L14 L15 | A2 L13 L16 bodies 5
fillet "Fillet20" radius 0.5 6 edges at (-9.47, 15.0618, 8.2) (-13.97, 11.78, 8.2) (-18.47, 15.0618, 8.2) (-13.97, 11.78, 9.2) (-9.47, 15.0618, 9.2) (-18.47, 15.0618, 9.2) on bodies 5
fillet "Fillet21" radius 6.5 3 edges at (-2.4593, 12.5235, -13.3) (18.7707, -33.9465, -13.3) (-26.2293, -33.9465, -13.3) on bodies 2
sketch "Sketch21" plane through (0, 0, 8.2) normal (0, 0, -1) x (1, 0, 0)
  arc A0 (0.3092, -0.4178) -> (0.3092, 0.4178) centre (0.0345, 0) ccw
  arc A1 (0.3092, 7.2022) -> (0.3092, 0.4178) centre (2.54, 3.81) ccw
  arc A2 (0.3092, 7.2022) -> (0.3092, 8.0378) centre (0.0345, 7.62) ccw
  arc A3 (0.3092, 14.8222) -> (0.3092, 8.0378) centre (2.54, 11.43) ccw
  arc A4 (0.3092, 14.8222) -> (0.3092, 15.6578) centre (0.0345, 15.24) ccw
  arc A5 (4.7708, 15.6578) -> (0.3092, 15.6578) centre (2.54, 19.05) ccw
  arc A6 (4.7708, 15.6578) -> (4.7708, 14.8222) centre (5.0455, 15.24) ccw
  arc A7 (4.7708, 8.0378) -> (4.7708, 14.8222) centre (2.54, 11.43) ccw
  arc A8 (4.7708, 8.0378) -> (4.7708, 7.2022) centre (5.0455, 7.62) ccw
  arc A9 (4.7708, 0.4178) -> (4.7708, 7.2022) centre (2.54, 3.81) ccw
  arc A10 (4.7708, 0.4178) -> (4.7708, -0.4178) centre (5.0455, 0) ccw
  arc A11 (0.3092, -0.4178) -> (4.7708, -0.4178) centre (2.54, -3.81) ccw
  line L0 (12.7, -5.08) -> (12.7, 17.78)
  line L1 (12.7, 17.78) -> (20.32, 17.78)
  line L2 (20.32, 17.78) -> (20.32, -5.08)
  line L3 (20.32, -5.08) -> (12.7, -5.08)
  circle A12 centre (1.27, -13.97) radius 3.75
  line L4 (-18.97, -18.5479) -> (-18.97, -11.28)
  line L5 (-18.97, -11.28) -> (-8.97, -11.28)
  line L6 (-8.97, -11.28) -> (-8.97, -18.5479)
  arc A13 (-7.9833, -20.05) -> (-8.97, -18.5479) centre (-9.97, -20.28) ccw
  line L7 (-7.9833, -20.05) -> (23.25, -20.05)
  arc A14 (23.25, -20.05) -> (26.25, -17.05) centre (23.25, -17.05) ccw
  line L8 (26.25, -17.05) -> (26.25, 32.5)
  circle A15 centre (22.5, 32.5) radius 3.75
  line L9 (26.25, 32.5) -> (26.25, 38.25)
  arc A16 (26.25, 38.25) -> (23.25, 41.25) centre (23.25, 38.25) ccw
  line L10 (23.25, 41.25) -> (-23.25, 41.25)
  arc A17 (-23.25, 41.25) -> (-26.25, 38.25) centre (-23.25, 38.25) ccw
  line L11 (-26.25, 38.25) -> (-26.25, 32.5)
  circle A18 centre (-22.5, 32.5) radius 3.75
  line L12 (-26.25, 32.5) -> (-26.25, -17.05)
  arc A19 (-26.25, -17.05) -> (-23.25, -20.05) centre (-23.25, -17.05) ccw
  line L13 (-23.25, -20.05) -> (-19.9567, -20.05)
  arc A20 (-18.97, -18.5479) -> (-19.9567, -20.05) centre (-17.97, -20.28) ccw
  line L14 (-9.47, -17.78) -> (-9.47, -11.78)
  line L15 (-9.47, -11.78) -> (-18.47, -11.78)
  line L16 (-18.47, -11.78) -> (-18.47, -17.78)
  line L17 (-18.47, -17.78) -> (-22.86, -17.78)
  line L18 (-22.86, -17.78) -> (-22.86, 17.78)
  line L19 (-22.86, 17.78) -> (-5.08, 17.78)
  line L20 (-5.08, 17.78) -> (-5.08, -17.78)
  line L21 (-5.08, -17.78) -> (-9.47, -17.78)
  line L22 (-17.97, 8.22) -> (-9.97, 8.22)
  line L23 (-9.97, 8.22) -> (-9.97, 16.22)
  line L24 (-9.97, 16.22) -> (-17.97, 16.22)
  line L25 (-17.97, 16.22) -> (-17.97, 8.22)
  line L26 (-13.97, 17.78) -> (-13.97, -11.28) construction
  line L27 (-9.97, 12.22) -> (-17.97, 12.22) construction
  point P0 (-13.97, 12.22)
  dimension "d192" = 8
  dimension "d193" = 30
  constraint horizontal L22
  constraint vertical L23
  constraint horizontal L24
  constraint vertical L25
  constraint midpoint L19 L26.start
  constraint midpoint L5 L26.end
  constraint equal L22 L25
  constraint midpoint L23 L27.start
  constraint midpoint L25 L27.end
  constraint midpoint L27 P0
  constraint coincident L26 P0
  measures "d192" distance of L23.end L24.end
  measures "d193" distance of L16.end L27
extrude "Extrude29" cut sketch "Sketch21" against normal blind 1 contours L22 L23 L24 L25 bodies 5
fillet "Fillet22" radius 0.5 8 edges at (-13.97, -16.22, 9.2) (-9.97, -12.22, 9.2) (-13.97, -8.22, 9.2) (-17.97, -12.22, 9.2) (-17.97, -12.22, 8.2) (-13.97, -8.22, 8.2) (-9.97, -12.22, 8.2) (-13.97, -16.22, 8.2) on bodies 5